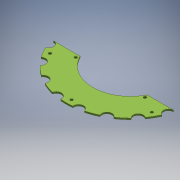
# Autodesk Inventor part: Board_Shape
Saved by Autodesk Inventor 2016 (Build 200138000, 138)
## iProperties
Created: 2015-08-05
Part Number: Board_Shape
Material: Generic
Document SubType Name: Modeling
Designer: 3DPrinterUser
Density: 1 g/cm^3
Appearance: Olive Green
Author: 3DPrinterUser
Autodesk Inventor part; units mm, degrees
ref_plane "YZ Plane" through (0, 0, 0) normal (1, 0, 0) x (0, 1, 0)
ref_plane "XZ Plane" through (0, 0, 0) normal (0, 1, 0) x (-1, 0, 0)
ref_plane "XY Plane" through (0, 0, 0) normal (0, 0, 1) x (1, 0, 0)
sketch "Sketch1" plane through (0, 0, 0) normal (0, 0, 1) x (1, 0, 0)
  circle A0 centre (-50.5576, -172.2408) radius 1.05 projected
  circle A1 centre (-57.0003, -171.3793) radius 1.05 projected
  circle A2 centre (45.6996, -106.0744) radius 1.05 construction
  circle A3 centre (52.1422, -106.9359) radius 1.05 construction
  arc A4 (-74.5492, -116.4853) -> (-70.0575, -105.3678) centre (-72.5241, -110.8373) ccw projected
  arc A5 (-74.5492, -116.4853) -> (-75.9551, -156.7439) centre (-2.429, -139.1576) ccw projected
  arc A6 (-72.2498, -168.1476) -> (-75.9551, -156.7439) centre (-74.3289, -162.5193) ccw projected
  arc A7 (-72.2498, -168.1476) -> (-65.5061, -180.8307) centre (-2.429, -139.1576) ccw projected
  arc A8 (-58.1239, -190.2794) -> (-65.5061, -180.8307) centre (-62.0026, -185.7016) ccw projected
  arc A9 (-58.1239, -190.2794) -> (-47.449, -199.8911) centre (-2.429, -139.1576) ccw projected
  arc A10 (-37.2804, -206.2451) -> (-47.449, -199.8911) centre (-42.4909, -203.27) ccw projected
  arc A11 (-37.2804, -206.2451) -> (-23.9619, -211.6262) centre (-2.429, -139.1576) ccw projected
  arc A12 (-12.2334, -214.1192) -> (-23.9619, -211.6262) centre (-18.1471, -213.1056) ccw projected
  arc A13 (-12.2334, -214.1192) -> (2.1224, -214.6205) centre (-2.429, -139.1576) ccw projected
  arc A14 (13.9963, -212.9517) -> (2.1224, -214.6205) centre (8.0925, -214.0219) ccw projected
  arc A15 (13.9963, -212.9517) -> (27.6578, -208.5128) centre (-2.429, -139.1576) ccw projected
  arc A16 (38.2448, -202.8836) -> (27.6578, -208.5128) centre (33.063, -205.9084) ccw projected
  arc A17 (38.2448, -202.8836) -> (49.5642, -194.0399) centre (-2.429, -139.1576) ccw projected
  arc A18 (57.5874, -185.1292) -> (49.5642, -194.0399) centre (53.7527, -189.7439) ccw projected
  arc A19 (57.5874, -185.1292) -> (65.1995, -172.9474) centre (-2.429, -139.1576) ccw projected
  arc A20 (69.6912, -161.8299) -> (65.1995, -172.9474) centre (67.6661, -167.4779) ccw projected
  arc A21 (69.6912, -161.8299) -> (71.0971, -121.5713) centre (-2.429, -139.1576) ccw projected
  arc A22 (67.3918, -110.1676) -> (71.0971, -121.5713) centre (69.4709, -115.7959) ccw projected
  arc A23 (67.3918, -110.1676) -> (60.648, -97.4845) centre (-2.429, -139.1576) ccw projected
  arc A24 (53.2659, -88.0358) -> (60.648, -97.4845) centre (57.1446, -92.6136) ccw projected
  arc A25 (53.2659, -88.0358) -> (42.591, -78.4241) centre (-2.429, -139.1576) ccw projected
  arc A26 (32.4224, -72.0701) -> (42.591, -78.4241) centre (37.6329, -75.0452) ccw projected
  arc A27 (32.4224, -72.0701) -> (19.1039, -66.689) centre (-2.429, -139.1576) ccw projected
  arc A28 (7.3754, -64.196) -> (19.1039, -66.689) centre (13.2891, -65.2096) ccw projected
  arc A29 (7.3754, -64.196) -> (-6.9804, -63.6947) centre (-2.429, -139.1576) ccw projected
  arc A30 (-18.8543, -65.3635) -> (-6.9804, -63.6947) centre (-12.9505, -64.2933) ccw projected
  arc A31 (-18.8543, -65.3635) -> (-32.5158, -69.8024) centre (-2.429, -139.1576) ccw projected
  arc A32 (-43.1028, -75.4316) -> (-32.5158, -69.8024) centre (-37.9211, -72.4068) ccw projected
  arc A33 (-43.1028, -75.4316) -> (-54.4222, -84.2753) centre (-2.429, -139.1576) ccw projected
  arc A34 (-62.4454, -93.186) -> (-54.4222, -84.2753) centre (-58.6108, -88.5713) ccw projected
  arc A35 (-62.4454, -93.186) -> (-70.0575, -105.3678) centre (-2.429, -139.1576) ccw projected
  circle A36 centre (-2.429, -139.1576) radius 44.3 projected
  circle A37 centre (67.8797, -130.1058) radius 1.3 projected
  circle A38 centre (44.0911, -152.2891) radius 1.3 projected
  circle A39 centre (-71.935, -125.2234) radius 1.3 projected
  circle A40 centre (-49.7517, -149.0121) radius 1.3 projected
  circle A41 centre (-72.7377, -148.2094) radius 1.3 projected
  circle A42 centre (-48.9491, -126.0261) radius 1.3 projected
  circle A43 centre (67.077, -153.0918) radius 1.3 projected
  circle A44 centre (44.8937, -129.3031) radius 1.3 projected
  circle A45 centre (55.9854, -141.1975) radius 11.5 projected
  circle A46 centre (-60.8434, -137.1177) radius 11.5 projected
  circle A47 centre (-61.4532, -102.2752) radius 1.55 projected
  circle A48 centre (-45.279, -84.3121) radius 1.55 projected
  circle A49 centre (-17.0455, -94.1726) radius 1.55 projected
  circle A50 centre (0, -69.6) radius 1.55 projected
  circle A51 centre (23.6436, -74.6256) radius 1.55 projected
  circle A52 centre (29.2209, -104.0069) radius 1.55 projected
  circle A53 centre (59.0241, -106.4824) radius 1.55 projected
  circle A54 centre (-63.8822, -171.8328) radius 1.55 projected
  circle A55 centre (-49.0005, -190.8805) radius 1.55 projected
  circle A56 centre (-28.5016, -203.6896) radius 1.55 projected
  circle A57 centre (37.6837, -164.2228) radius 1.55 projected
  circle A58 centre (26.6918, -176.4305) radius 1.55 projected
  circle A59 centre (12.1875, -184.1426) radius 1.55 projected
  circle A60 centre (-4.0798, -186.4288) radius 1.55 projected
  circle A61 centre (-4.858, -208.7152) radius 1.55 projected
  circle A62 centre (19.0786, -205.3511) radius 1.55 projected
  circle A63 centre (40.421, -194.0032) radius 1.55 projected
  circle A64 centre (56.5951, -176.04) radius 1.55 projected
  circle A65 centre (-20.1479, -183.0134) radius 1.55 projected
  circle A66 centre (-34.0789, -174.3084) radius 1.55 projected
  circle A67 centre (-44.1924, -161.3636) radius 1.55 projected
  circle A68 centre (39.3344, -116.9516) radius 1.55 projected
  circle A69 centre (44.1425, -87.4347) radius 1.55 projected
  circle A70 centre (15.2899, -95.3018) radius 1.55 projected
  circle A71 centre (-0.7783, -91.8864) radius 1.55 projected
  circle A72 centre (-23.9366, -72.9641) radius 1.55 projected
  circle A73 centre (-31.5498, -101.8847) radius 1.55 projected
  circle A74 centre (-42.5417, -114.0924) radius 1.55 projected
  line L0 (-60.8434, 0) -> (-2.429, 0) construction
  line L1 (-72.5241, -104.8373) -> (25.5819, -104.8373)
  line L2 (69.4709, -109.7959) -> (-35.601, -109.7959)
  point P0 (0, 0)
  constraints: 6 end point, 4 point on circle, 2 parallel, 2 tangent, 1 horizontal
extrude "Extrusion1" add sketch "Sketch1" along normal blind 1.75 contours A0 | A1 | A4 A35 L1 A36 L2 A23 A22 A21 A20 A19 A18 A17 A16 A15 A14 A13 A12 A11 A10 A9 A8 A7 A6 A5 | A35 A34 A33 A32 A31 A30 A29 A28 A27 A26 A25 A24 A23 L2 A36 L1 | L1 A36 L2 | A36 L1 | L2 A36 | A37 | A38 | A39 | A40 | A41 | A42 | A43 | A44 | A45 | A46 | A54 | A55 | A56 | A57 | A58 | A59 | A60 | A61 | A62 | A63 | A64 | A65 | A66 | A67
sketch "Sketch2" plane through (0, 0, 1.75) normal (0, 0, 1) x (1, 0, 0)
  circle A0 centre (29.2209, -104.0069) radius 1.55 projected
  circle A1 centre (44.1425, -87.4347) radius 1.55 projected
  circle A2 centre (23.6436, -74.6256) radius 1.55 projected
  circle A3 centre (15.2899, -95.3018) radius 1.55 projected
  circle A4 centre (-17.0455, -94.1726) radius 1.55 projected
  circle A5 centre (-23.9366, -72.9641) radius 1.55 projected
  circle A6 centre (-45.279, -84.3121) radius 1.55 projected
  circle A7 centre (-31.5498, -101.8847) radius 1.55 projected
  circle A8 centre (-0.7783, -91.8864) radius 1.55 projected
  point P0 (0, 0)
extrude "Extrusion2" add sketch "Sketch2" against normal up to surface (1.75 mm away)
equation "\"d0\" = board_height"
equation "\"d2\" = board_height"
equation "\"board_height\" = 1.75"
body "Solid1"
